Autodesk Inventor part; units mm, degrees
(part 2 of 2)
sketch "Sketch2" plane through (0.5941, 47.0928, 3) normal (0, 0, 1) x (0.9921226, 0.125271, 0)
  arc A0 (-433.0678, -42.3519) -> (-429.5322, -42.3519) centre (-431.3, -40.5842) ccw projected
  line L0 (-429.5322, -42.3519) -> (-377.3059, 9.8744) projected
  arc A1 (-377.3059, 9.8744) -> (-376.5737, 11.6421) centre (-379.0737, 11.6421) ccw projected
  line L1 (-376.5737, 11.6421) -> (-376.5737, 21.1698) projected
  arc A2 (-376.5737, 21.1698) -> (-376.987, 22.5467) centre (-379.0737, 21.1698) ccw projected
  line L2 (-376.987, 22.5467) -> (-382.6099, 31.0681) projected
  arc A3 (-382.6099, 31.0681) -> (-382.6649, 31.1498) centre (-386.85, 28.2703) ccw projected
  arc A4 (-382.6649, 31.1498) -> (-384.7245, 32.2327) centre (-384.7245, 29.7327) ccw projected
  line L3 (-384.7245, 32.2327) -> (-389.0363, 32.2327) projected
  arc A5 (-389.0363, 32.2327) -> (-390.804, 31.5005) centre (-389.0363, 29.7327) ccw projected
  line L4 (-390.804, 31.5005) -> (-403.1421, 19.1624) projected
  arc A6 (-403.1421, 19.1624) -> (-404.63, 15.5703) centre (-399.55, 15.5703) ccw projected
  line L5 (-404.63, 15.5703) -> (-404.63, 4.385) projected
  arc A7 (-412.0695, -13.5755) -> (-404.63, 4.385) centre (-430.03, 4.385) ccw projected
  line L6 (-412.0695, -13.5755) -> (-435.1891, -36.6951) projected
  arc A8 (-435.1891, -36.6951) -> (-435.1891, -40.2306) centre (-433.4213, -38.4628) ccw projected
  line L7 (-435.1891, -40.2306) -> (-433.0678, -42.3519) projected
  arc A9 (-380.8126, 9.8325) -> (-383.0046, 12.0246) centre (-381.9086, 10.9286) ccw projected
  line L8 (-380.8126, 9.8325) -> (-394.283, -3.6378) projected
  arc A10 (-396.475, -1.4458) -> (-394.283, -3.6378) centre (-395.379, -2.5418) ccw projected
  line L9 (-396.475, -1.4458) -> (-383.0046, 12.0246) projected
  circle A11 centre (-404.3592, -11.5221) radius 2.159 projected
  arc A12 (-432.396, -37.3668) -> (-430.204, -39.5589) centre (-431.3, -38.4628) ccw projected
  line L10 (-432.396, -37.3668) -> (-414.4355, -19.4063) projected
  arc A13 (-412.2435, -21.5984) -> (-414.4355, -19.4063) centre (-413.3395, -20.5023) ccw projected
  line L11 (-412.2435, -21.5984) -> (-430.204, -39.5589) projected
  circle A14 centre (-393.2, 21.9203) radius 2.159 projected
  circle A15 centre (-399.55, 15.5703) radius 2.159 projected
  circle A16 centre (-386.85, 28.2703) radius 2.159 projected
  line L12 (-384.993, 29.2327) -> (-379.5737, 21.0197)
  line L13 (-379.5737, 21.0197) -> (-379.5737, 11.8492)
  line L14 (-379.5737, 11.8492) -> (-431.3, -39.8771)
  line L15 (-431.3, -39.8771) -> (-432.7142, -38.4628)
  line L16 (-432.7142, -38.4628) -> (-409.9482, -15.6968)
  arc A17 (-409.9482, -15.6968) -> (-401.63, 4.385) centre (-430.03, 4.385) ccw
  line L17 (-401.63, 4.385) -> (-401.63, 15.5703)
  arc A18 (-401.0208, 17.0411) -> (-401.63, 15.5703) centre (-399.55, 15.5703) ccw
  line L18 (-401.0208, 17.0411) -> (-388.8292, 29.2327)
  line L19 (-388.8292, 29.2327) -> (-384.993, 29.2327)
  arc A19 (-378.6913, 7.7112) -> (-385.1259, 14.1459) centre (-381.9086, 10.9286) ccw
  line L20 (-378.6913, 7.7112) -> (-392.1616, -5.7592)
  arc A20 (-398.5963, 0.6755) -> (-392.1616, -5.7592) centre (-395.379, -2.5418) ccw
  line L21 (-398.5963, 0.6755) -> (-385.1259, 14.1459)
  circle A21 centre (-404.3592, -11.5221) radius 5.159
  circle A22 centre (-399.55, 15.5703) radius 5.159
  circle A23 centre (-393.2, 21.9203) radius 5.159
  circle A24 centre (-386.85, 28.2703) radius 5.159
  circle A25 centre (-399.9958, 1.7447) radius 1.75
  point P0 (-6.4888, -46.6475)
  point P1 (-379.5737, 14.8338)
  point P2 (-382.5137, 25.4753)
  point P3 (-388.2286, 23.2989)
  point P4 (-394.5786, 16.9489)
  point P5 (-401.63, 10.8492)
  point P6 (-401.7391, 1.898)
  point P7 (-398.7134, 0.554)
  dimension "d15" = 3
  dimension "d16" = 3
  dimension "d17" = 3
  dimension "d18" = 3
  dimension "d19" = 3.5
  constraints: 20 end point, 9 centre point, 8 point on circle, 2 coincident, 2 equal radius, 2 tangent, 12 other
  measures "d15" distance between parallel lines of L2 L12
  measures "d16" distance between parallel lines of L9 L21
  measures "d17" radial gap between concentric circles of A11 A21
  measures "d18" radial gap between concentric circles of A15 A22
  measures "d19" diameter of A25
extrude "Extrusion2" cut sketch "Sketch2" against normal blind 2 contours A19 L21 A20 A25 A17 L17 A22 A23 A24 L12 L13 | A25
fillet "Fillet3" radius 1.75 6 edges at (-378.6227, 20.3974, 2) (-377.8478, 14.2602, 2) (-382.0977, 24.4496, 2) (-387.4949, 21.5744, 2) (-392.9994, 14.479, 2) (-399.2312, 7.544, 2)
body "Solid1"
